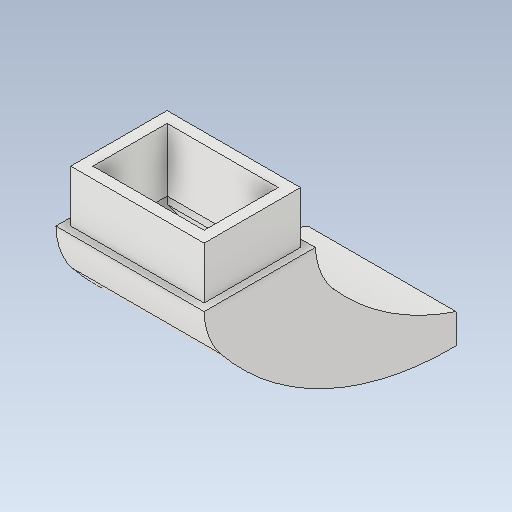
# Autodesk Inventor part: 45_dysza chłodząca
Saved by Autodesk Inventor 2020.2 (Build 242310000, 310)
## iProperties
Created: 2017-11-19
Part Number: 45_dysza chłodząca
Material: Ogólny
Document SubType Name: Modeling
Designer: Haras
Density: 1 g/cm^3
Appearance: Śnieg
Author: Haras
Autodesk Inventor part; units mm, degrees
ref_plane "YZ Plane" through (0, 0, 0) normal (1, 0, 0) x (0, 1, 0)
ref_plane "XZ Plane" through (0, 0, 0) normal (0, 1, 0) x (-1, 0, 0)
ref_plane "XY Plane" through (0, 0, 0) normal (0, 0, 1) x (1, 0, 0)
sketch "Szkic1" plane through (0, 0, 0) normal (0, 1, 0) x (-1, 0, 0)
  line L0 (9, 6.5) -> (-9, 6.5)
  line L1 (-9, 6.5) -> (-9, -6.5)
  line L2 (-9, -6.5) -> (9, -6.5)
  line L3 (9, -6.5) -> (9, 6.5)
  line L4 (9, 0) -> (0, 0) construction
  line L5 (0, 0) -> (0, -6.5) construction
  dimension "d0" = 13
  dimension "d1" = 18
  constraints: 12 end point, 2 horizontal, 2 midpoint, 2 parallel, 1 perpendicular, 1 vertical
  measures "d0" distance of L2.end L0.start
  measures "d1" distance of L1.end L2.end
extrude "Wyciągnięcie proste1" add sketch "Szkic1" along normal blind 7
sketch "Szkic2" plane through (0, 0, 0) normal (0, -1, 0) x (1, 0, 0)
  line L0 (-10, 7.5) -> (10, 7.5)
  line L1 (10, 7.5) -> (10, -7.5)
  line L2 (10, -7.5) -> (-10, -7.5)
  line L3 (-10, -7.5) -> (-10, 7.5)
  line L4 (0, 7.5) -> (0, 0) construction
  line L5 (0, 0) -> (10, 0) construction
  dimension "d4" = 20
  dimension "d5" = 15
  constraints: 12 end point, 2 horizontal, 2 midpoint, 2 parallel, 1 perpendicular, 1 vertical
  measures "d4" distance of L0.start L0.end
  measures "d5" distance of L0.end L1.end
extrude "Wyciągnięcie proste2" add sketch "Szkic2" along normal blind 3
sketch "Szkic3" plane through (10, 0, 7.5) normal (1, 0, 0) x (0, 0, -1)
  line L0 (0, 0) -> (0, -3) projected
  arc A0 (0, -3) -> (34, -21) centre (33.4095, 18.9956) ccw
  line L1 (1, 7) -> (14, 7) projected
  line L2 (0, -3) -> (15, -3) projected
  arc A1 (15, -3) -> (34, -17) centre (45.9271, 19.0797) ccw
  line L3 (34, -17) -> (34, -21)
  line L4 (15, 0) -> (15, -3) projected
  line L5 (0, -3) -> (15, -3)
  point P0 (7.5, 0)
  dimension "d10" = 34
  dimension "d11" = 40
  dimension "d12" = 28
  dimension "d13" = 4
  dimension "d14" = 38
  constraints: 4 end point, 4 point on circle, 2 centre point, 1 horizontal, 1 vertical, 1 vertical alignment
  measures "d10" distance from line of L3.end L0
  measures "d11" radius of A0
  measures "d12" distance from line of L3.end L1
  measures "d13" distance of L3.end L3.start
  measures "d14" radius of A1
extrude "Wyciągnięcie proste3" add sketch "Szkic3" against normal up to surface (20 mm away)
shell "Skorupa1" thickness 1.5 removed faces 2 at (-3, 7, 2.1667) at (-3.3333, -19.6667, -26.5)
fillet "Zaokrąglenie1" radius 10 2 edges at (0, -3, -7.5) (0, -3, 7.5)
chamfer "Faza1" distance 1 angle 45 1 edges at (0, -19.4998, -26.5)
